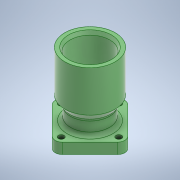
# Autodesk Inventor part: 22M_PEEP_Port_Female_Green
Saved by Autodesk Inventor 2020 (Build 240168000, 168)
## iProperties
Created: 2021-05-21
Part Number: 22M_PEEP_Port_Female_Green
Material: Generic
Document SubType Name: Modeling
Designer: Workshop
Density: 1 g/cm^3
Appearance: Smooth - Dark Forest Green
Author: Workshop
Autodesk Inventor part; units mm, degrees
ref_plane "YZ Plane" through (0, 0, 0) normal (1, 0, 0) x (0, 1, 0)
ref_plane "XZ Plane" through (0, 0, 0) normal (0, 1, 0) x (-1, 0, 0)
ref_plane "XY Plane" through (0, 0, 0) normal (0, 0, 1) x (1, 0, 0)
sketch "Sketch1" plane through (0, 0, 0) normal (0, 0, 1) x (1, 0, 0)
  line L0 (0, 11.1253) -> (0, 14.1253)
  line L1 (0, 14.1253) -> (23, 14.1253)
  line L2 (23, 14.1253) -> (27.51, 10.8753)
  line L3 (27.51, 10.8753) -> (35.51, 10.8753)
  line L4 (35.51, 10.8753) -> (35.51, 25)
  line L5 (35.51, 25) -> (41.51, 25)
  line L6 (41.51, 25) -> (41.51, 10)
  line L7 (38.901, 7.8753) -> (26.5417, 7.8753)
  line L8 (26.5417, 7.8753) -> (22.0317, 11.1253)
  line L9 (0, 11.1253) -> (22.0317, 11.1253)
  line L10 (38.901, 7.8753) -> (41.51, 10)
  line L11 (-8.302, 0) -> (49.812, 0) projected
  point P0 (0, 0)
  dimension "d0" = 3
  dimension "d1" = 23
  dimension "d2" = 6
  dimension "d3" = 11.1253
  dimension "d4" = 4.51
  dimension "d5" = 3.25
  dimension "d6" = 3
  dimension "d7" = 8
  dimension "d8" = 25
  dimension "d9" = 10
  dimension "d11" = 3
  dimension "d12" = 2.609
  constraints: 22 end point, 4 perpendicular, 3 parallel, 1 horizontal, 1 vertical, 1 vertical alignment
  measures "d0" distance of L0.start L0.end
  measures "d1" distance of L0.end L1.end
  measures "d2" distance of L4.end L5.end
  measures "d3" distance of point (0, 0) L0.start
  measures "d4" horizontal distance of L2.end L1.end
  measures "d5" vertical distance of L2.end L1.end
  measures "d6" distance between parallel lines of L7 L3
  measures "d7" distance of L2.end L3.end
  measures "d8" distance from line of point (0, 0) L5
  measures "d9" vertical distance of point (0, 0) L6.end
  measures "d11" distance between parallel lines of L8 L2
  measures "d12" horizontal distance of L6.end L7.start
revolve "Revolution1" add sketch "Sketch1" angle 360 about axis through (-10, 0, 0) along (1, 0, 0)
chamfer "Chamfer1" distance 0.875 distance2 2 1 edges at (0, -11.1253, 0) measured on face at (0, -11.6253, 0)
fillet "Fillet1" radius 2 1 edges at (35.51, -10.8753, 0)
fillet "Fillet2" radius 2 1 edges at (27.51, -10.8753, 0)
sketch "Sketch2" plane through (41.51, 0, 0) normal (1, 0, 0) x (0, 0, -1)
  circle A0 centre (0, -16.125) radius 1.6
  circle A1 centre (0, 0) radius 25 projected
  circle A2 centre (16.125, 0) radius 1.6
  circle A3 centre (0, 16.125) radius 1.6
  circle A4 centre (-16.125, 0) radius 1.6
  line L0 (0, 21.1425) -> (21.1425, 0)
  line L1 (21.1425, 0) -> (0, -21.1425)
  line L2 (0, -21.1425) -> (-21.1425, 0)
  line L3 (-21.1425, 0) -> (0, 21.1425)
  line L4 (0, 21.1425) -> (0, -21.1425) construction
  line L5 (21.1425, 0) -> (-21.1425, 0) construction
  point P0 (0, 0)
  dimension "d19" = 3.2
  dimension "d20" = 16.125
  dimension "d23" = 360
  dimension "d25" = 29.9
  constraints: 12 end point, 4 centre point, 4 midpoint, 2 parallel, 2 perpendicular, 2 vertical alignment, 1 horizontal alignment, 9 other
  measures "d19" diameter of A0
  measures "d20" distance of point (0, 0) A0.centre
  measures "d25" distance between parallel lines of L2 L0
extrude "Extrusion1" cut sketch "Sketch2" against normal blind 10
fillet "Fillet3" radius 4 4 edges at (38.51, 21.1425, 0) (38.51, 0, -21.1425) (38.51, 0, 21.1425) (38.51, -21.1425, 0)
fillet "Fillet4" radius 2 1 edges at (22.0317, -11.1253, 0)
body "Solid1"
